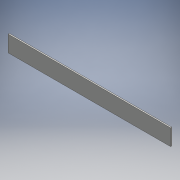
# Autodesk Inventor part: bed_wall
Saved by Autodesk Inventor 2016 (Build 200138000, 138)
## iProperties
Created: 2015-09-03
Part Number: bed_wall
Material: Generic
Document SubType Name: Modeling
Designer: oscar
Density: 1 g/cm^3
Appearance: Default
Author: oscar
Autodesk Inventor part; units mm, degrees
ref_plane "YZ Plane" through (0, 0, 0) normal (1, 0, 0) x (0, 1, 0)
ref_plane "XZ Plane" through (0, 0, 0) normal (0, 1, 0) x (-1, 0, 0)
ref_plane "XY Plane" through (0, 0, 0) normal (0, 0, 1) x (1, 0, 0)
sketch "Sketch1" plane through (0, 0, 0) normal (0, 1, 0) x (-1, 0, 0)
  line L0 (0, 0) -> (800, 0)
  line L1 (800, 0) -> (800, 80)
  line L2 (800, 80) -> (0, 80)
  line L3 (0, 80) -> (0, 0)
  dimension "d0" = 80
  dimension "d1" = 800
  constraints: 8 end point, 2 parallel, 1 horizontal, 1 perpendicular
  measures "d0" distance of L0.end L1.end
  measures "d1" distance of L1.end L2.end
extrude "Extrusion1" add sketch "Sketch1" along normal blind 6
body "Solid1"
